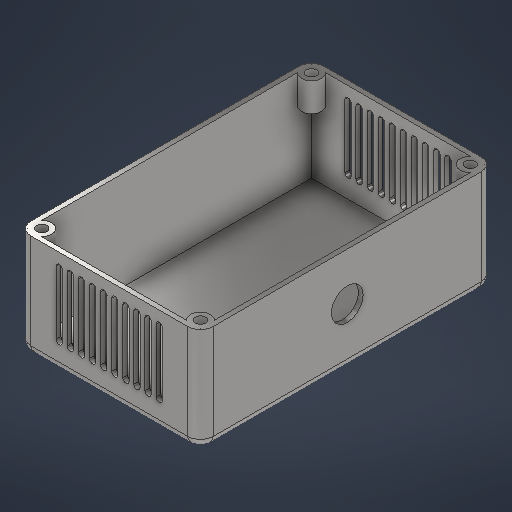
# Autodesk Inventor part: base mbg
Saved by Autodesk Inventor 2026.3 (Build 303398000, 398)
## iProperties
Created: 2026-06-09
Part Number: base mbg
Material: Stainless Steel
Document SubType Name: Modeling
Designer: ilyas
Density: 8 g/cm^3
Appearance: Semi-Polished
Author: ilyas
Autodesk Inventor part; units mm, degrees
ref_plane "YZ Plane" through (0, 0, 0) normal (1, 0, 0) x (0, 1, 0)
ref_plane "XZ Plane" through (0, 0, 0) normal (0, 1, 0) x (-1, 0, 0)
ref_plane "XY Plane" through (0, 0, 0) normal (0, 0, 1) x (1, 0, 0)
sketch "Sketch1" plane through (0, 0, 0) normal (0, 1, 0) x (-1, 0, 0)
  line L0 (-57.5, 92.5) -> (57.5, 92.5)
  line L1 (57.5, 92.5) -> (57.5, -92.5)
  line L2 (57.5, -92.5) -> (-57.5, -92.5)
  line L3 (-57.5, -92.5) -> (-57.5, 92.5)
  line L4 (-57.5, 92.5) -> (57.5, -92.5) construction
  line L5 (57.5, 92.5) -> (-57.5, -92.5) construction
  point P0 (0, 0)
  dimension "d0" = 115
  dimension "d1" = 185
  constraints: 12 end point, 2 midpoint, 2 parallel, 1 horizontal, 1 perpendicular
  measures "d0" distance of L1.end L2.end
  measures "d1" distance of L0.end L1.end
extrude "Extrusion1" add sketch "Sketch1" along normal blind 65
sketch "Sketch2" plane through (0, 65, 0) normal (0, 1, 0) x (1, 0, 0)
  line L0 (-57.5, 92.5) -> (-57.5, -92.5) projected
  line L1 (-57.5, -92.5) -> (-42.5, -92.5)
  line L2 (-42.5, -92.5) -> (-42.5, -77.5)
  line L3 (-42.5, -77.5) -> (-57.5, -77.5)
  line L4 (-57.5, -77.5) -> (-57.5, -92.5)
  line L5 (-57.5, 92.5) -> (-42.5, 92.5)
  line L6 (-42.5, 92.5) -> (-42.5, 77.5)
  line L7 (-42.5, 77.5) -> (-57.5, 77.5)
  line L8 (-57.5, 77.5) -> (-57.5, 92.5)
  line L9 (-57.5, -92.5) -> (57.5, -92.5) projected
  line L10 (57.5, -92.5) -> (42.5, -92.5)
  line L11 (42.5, -92.5) -> (42.5, -77.5)
  line L12 (42.5, -77.5) -> (57.5, -77.5)
  line L13 (57.5, -77.5) -> (57.5, -92.5)
  line L14 (57.5, 92.5) -> (42.5, 92.5)
  line L15 (42.5, 92.5) -> (42.5, 77.5)
  line L16 (42.5, 77.5) -> (57.5, 77.5)
  line L17 (57.5, 77.5) -> (57.5, 92.5)
  line L18 (-42.5, -92.5) -> (-57.5, -77.5)
  line L19 (-42.5, -77.5) -> (-57.5, -92.5)
  line L20 (-42.5, 77.5) -> (-57.5, 92.5)
  line L21 (-57.5, 77.5) -> (-42.5, 92.5)
  line L22 (42.5, 77.5) -> (57.5, 92.5)
  line L23 (57.5, 77.5) -> (42.5, 92.5)
  line L24 (57.5, -92.5) -> (42.5, -77.5)
  line L25 (42.5, -92.5) -> (57.5, -77.5)
  point P0 (0, 0)
  point P1 (-50, -85)
  point P2 (-50, 85)
  point P3 (50, 85)
  point P4 (50, -85)
  dimension "d6" = 15
  dimension "d7" = 15
  dimension "d8" = 15
  dimension "d9" = 15
  dimension "d10" = 15
  dimension "d11" = 15
  dimension "d12" = 15
  dimension "d13" = 15
  constraints: 48 end point, 8 parallel, 4 horizontal, 4 midpoint, 4 perpendicular, 1 point on line
  measures "d6" distance of L3.end L2.end
  measures "d7" distance of L2.end L1.end
  measures "d8" distance of L6.end L7.end
  measures "d9" distance of L5.end L6.end
  measures "d10" distance of L11.end L12.end
  measures "d11" distance of L10.end L11.end
  measures "d12" distance of L16.end L15.end
  measures "d13" distance of L15.end L14.end
hole "Hole1" at (-50, 65, 85) at (-50, 65, -85) at (50, 65, -85) at (50, 65, 85) direction (0, -1, 0) diameter 6.576 depth 15
shell "Shell2" thickness 3 removed faces 1 at (-16.1573, 65, -27.3629)
fillet "Fillet2" radius 8 4 edges at (57.5, 32.5, 92.5) (-57.5, 32.5, 92.5) (57.5, 32.5, -92.5) (-57.5, 32.5, -92.5)
fillet "Fillet3" radius 5 8 edges at (55.1569, 0, -90.1569) (0, 0, -92.5) (-55.1569, 0, -90.1569) (-57.5, 0, 0) (-55.1569, 0, 90.1569) (0, 0, 92.5) (55.1569, 0, 90.1569) (57.5, 0, 0)
sketch "Sketch3" plane through (-49.5, 65, 92.5) normal (0, 0, 1) x (1, 0, 0)
  line L0 (23, -48.5) -> (23, -8.5)
  line L1 (27, -8.5) -> (27, -48.5)
  arc A0 (23, -48.5) -> (27, -48.5) centre (25, -48.5) ccw
  arc A1 (27, -8.5) -> (23, -8.5) centre (25, -8.5) ccw
  line L2 (30, -48.5) -> (30, -8.5)
  line L3 (34, -8.5) -> (34, -48.5)
  arc A2 (30, -48.5) -> (34, -48.5) centre (32, -48.5) ccw
  arc A3 (34, -8.5) -> (30, -8.5) centre (32, -8.5) ccw
  line L4 (37, -48.5) -> (37, -8.5)
  line L5 (41, -8.5) -> (41, -48.5)
  arc A4 (37, -48.5) -> (41, -48.5) centre (39, -48.5) ccw
  arc A5 (41, -8.5) -> (37, -8.5) centre (39, -8.5) ccw
  line L6 (44, -48.5) -> (44, -8.5)
  line L7 (48, -8.5) -> (48, -48.5)
  arc A6 (44, -48.5) -> (48, -48.5) centre (46, -48.5) ccw
  arc A7 (48, -8.5) -> (44, -8.5) centre (46, -8.5) ccw
  line L8 (51, -48.5) -> (51, -8.5)
  line L9 (55, -8.5) -> (55, -48.5)
  arc A8 (51, -48.5) -> (55, -48.5) centre (53, -48.5) ccw
  arc A9 (55, -8.5) -> (51, -8.5) centre (53, -8.5) ccw
  line L10 (58, -48.5) -> (58, -8.5)
  line L11 (62, -8.5) -> (62, -48.5)
  arc A10 (58, -48.5) -> (62, -48.5) centre (60, -48.5) ccw
  arc A11 (62, -8.5) -> (58, -8.5) centre (60, -8.5) ccw
  line L12 (65, -48.5) -> (65, -8.5)
  line L13 (69, -8.5) -> (69, -48.5)
  arc A12 (65, -48.5) -> (69, -48.5) centre (67, -48.5) ccw
  arc A13 (69, -8.5) -> (65, -8.5) centre (67, -8.5) ccw
  line L14 (72, -48.5) -> (72, -8.5)
  line L15 (76, -8.5) -> (76, -48.5)
  arc A14 (72, -48.5) -> (76, -48.5) centre (74, -48.5) ccw
  arc A15 (76, -8.5) -> (72, -8.5) centre (74, -8.5) ccw
  line L16 (79, -48.5) -> (79, -8.6)
  line L17 (83, -8.6) -> (83, -48.5)
  arc A16 (79, -48.5) -> (83, -48.5) centre (81, -48.5) ccw
  arc A17 (83, -8.6) -> (79, -8.6) centre (81, -8.6) ccw
  line L18 (16, -48.5) -> (16, -8.5)
  line L19 (20, -8.5) -> (20, -48.5)
  arc A18 (16, -48.5) -> (20, -48.5) centre (18, -48.5) ccw
  arc A19 (20, -8.5) -> (16, -8.5) centre (18, -8.5) ccw
  line L20 (99, -60) -> (0, -60) projected
  line L21 (0, -60) -> (0, 0) projected
  line L22 (0, 0) -> (99, 0) projected
  point P0 (49.5, -65)
  dimension "d41" = 7
  dimension "d42" = 18
  dimension "d43" = 7
  dimension "d44" = 7
  dimension "d45" = 7
  dimension "d46" = 7
  dimension "d48" = 11.5
  dimension "d49" = 11.5
  dimension "d50" = 11.5
  dimension "d52" = 11.5
  dimension "d53" = 7
  dimension "d54" = 8.5
  dimension "d55" = 8.5
  dimension "d56" = 11.5
  dimension "d57" = 8.5
  dimension "d58" = 7
  dimension "d59" = 7
  dimension "d60" = 11.5
  dimension "d61" = 7
  dimension "d62" = 11.5
  dimension "d63" = 8.6
  constraints: 40 end point, 40 point on circle, 40 tangent, 20 centre point, 10 equal radius, 10 parallel
  measures "d41" distance of A0.centre A18.centre
  measures "d42" distance from line of L21 A19.centre
  measures "d43" distance of A1.centre A3.centre
  measures "d44" distance of A2.centre A4.centre
  measures "d45" distance of A5.centre A7.centre
  measures "d46" distance of A6.centre A8.centre
  measures "d48" distance from line of L20 A18.centre
  measures "d49" distance from line of L20 A4.centre
  measures "d50" distance from line of L20 A8.centre
  measures "d52" distance from line of L20 A10.centre
  measures "d53" distance of A9.centre A11.centre
  measures "d54" distance from line of L22 A9.centre
  measures "d55" distance from line of L22 A11.centre
  measures "d56" distance from line of L20 A12.centre
  measures "d57" distance from line of L22 A13.centre
  measures "d58" distance of A10.centre A12.centre
  measures "d59" distance of A12.centre A14.centre
  measures "d60" distance from line of L20 A14.centre
  measures "d61" horizontal distance of A15.centre A17.centre
  measures "d62" distance from line of L20 A16.centre
  measures "d63" distance from line of L22 A17.centre
sketch "Sketch4" plane through (49.5, 65, -92.5) normal (0, 0, -1) x (-1, 0, 0)
  point P0 (49.5, -65)
extrude "Extrusion2" cut sketch "Sketch3" against normal through all
sketch "Sketch5" plane through (57.5, 65, 84.5) normal (1, 0, 0) x (0, 0, -1)
  line L0 (0, 0) -> (169, 0) projected
  line L1 (169, 0) -> (169, -60) projected
  line L2 (169, -60) -> (169, 0)
  line L3 (0, -60) -> (169, -60) projected
  circle A0 centre (84.5, -30) radius 10
  point P0 (84.5, -65)
  dimension "d66" = 20
  constraints: 2 end point, 1 centre point, 1 collinear
  measures "d66" diameter of A0
extrude "Extrusion3" cut sketch "Sketch5" against normal blind 10
body "Solid1"
